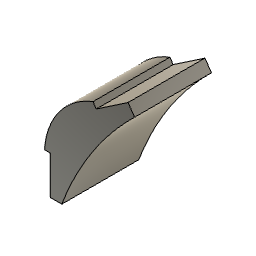
corner_rearmost v1 (Autodesk Fusion 360 design; units mm, degrees)
Autodesk Fusion 360 part; units mm, degrees
sketch "Rear Most Corner" plane through (0, 0, 0) normal (0, 1, 0) x (1, 0, 0)
  circle A0 centre (23.1977, -483.5644) radius 25 construction
  line L0 (14.257, -506.911) -> (24.7715, -514.0339) construction
  line L1 (407.957, -773.6165) -> (14.257, -506.911) construction
  line L2 (-1.7526, -485.14) -> (-1.7526, -472.44) construction
  line L3 (24.7715, -514.0339) -> (14.257, -506.911) construction
  line L4 (14.257, -506.911) -> (15.3255, -505.3338)
  line L5 (15.3255, -505.3338) -> (25.84, -512.4567)
  line L6 (25.84, -512.4567) -> (24.7715, -514.0339) construction
  line L7 (-1.7526, -485.14) -> (0.1524, -485.14)
  line L8 (0.1524, -485.14) -> (0.1524, -472.44)
  line L9 (0.1524, -472.44) -> (-1.7526, -472.44) construction
  line L10 (-1.7526, -472.44) -> (-1.7526, -485.14) construction
  line L11 (-1.7526, -485.14) -> (0.1524, -485.14)
  line L12 (14.257, -506.911) -> (15.3255, -505.3338)
  arc A1 (-1.7526, -485.14) -> (14.257, -506.911) centre (23.1977, -483.5644) ccw
  line L13 (25.84, -512.4567) -> (27.9768, -509.3024)
  line L14 (0.1524, -472.44) -> (3.9624, -472.44)
  line L15 (3.0571, -498.3751) -> (23.1977, -483.5644) construction
  arc A2 (3.9624, -472.44) -> (27.9768, -509.3024) centre (97.8219, -437.5475) ccw
  point P0 (13.1274, -490.9697)
extrude "Extrude1" add sketch "Rear Most Corner" along normal blind 25.4
